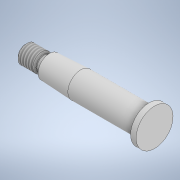
# Autodesk Inventor part: Палец_ребрышко
Saved by Autodesk Inventor 2021 (Build 250183000, 183)
## iProperties
Created: 2023-04-14
Part Number: Палец_ребрышко
Material: Типовые
Document SubType Name: Modeling
Designer: gdevc
Density: 1 g/cm^3
Appearance: По умолчанию
Author: gdevc
Autodesk Inventor part; units mm, degrees
ref_plane "YZ Plane" through (0, 0, 0) normal (1, 0, 0) x (0, 1, 0)
ref_plane "XZ Plane" through (0, 0, 0) normal (0, 1, 0) x (-1, 0, 0)
ref_plane "XY Plane" through (0, 0, 0) normal (0, 0, 1) x (1, 0, 0)
sketch "Эскиз1" plane through (0, 0, 0) normal (0, 0, 1) x (1, 0, 0)
  line L0 (0, 0) -> (0, 5)
  line L1 (0, 5) -> (10, 5)
  line L2 (10, 5) -> (10, 4)
  line L3 (10, 4) -> (13, 4)
  line L4 (13, 4) -> (13, 6.15)
  line L5 (13, 6.15) -> (30, 7)
  line L6 (30, 7) -> (67, 7)
  line L7 (67, 7) -> (67, 10)
  line L8 (67, 10) -> (70, 10)
  line L9 (70, 10) -> (70, 0)
  line L10 (0, 0) -> (70, 0)
  dimension "d0" = 10
  dimension "d1" = 12.3
  dimension "d2" = 14
  dimension "d3" = 10
  dimension "d4" = 3
  dimension "d5" = 20
  dimension "d6" = 8
  dimension "d7" = 60
  dimension "d8" = 3
  dimension "d9" = 20
  constraints: 22 end point, 5 perpendicular, 4 vertical, 1 horizontal
  measures "d0" diameter of L1 L10
  measures "d1" diameter of L4.end L10
  measures "d2" diameter of L5.end L10
  measures "d3" distance of L0.end L1.end
  measures "d4" distance of L2.end L3.end
  measures "d5" distance from line of L5.end L2
  measures "d6" diameter of L3 L10
  measures "d7" distance between parallel lines of L9 L2
  measures "d8" distance between parallel lines of L9 L7
  measures "d9" diameter of L8 L10
revolve "Вращение1" add sketch "Эскиз1" angle 360 about axis through (0, 0, 0) along (1, 0, 0)
thread "Резьба1" size "M10x1.5" class "6g" standard "ISO Metric profile" length 18
chamfer "Фаска1" distance 1 angle 45 2 edges at (0, -5, 0) (10, -5, 0)
fillet "Сопряжение1" radius 0.5 2 edges at (10, -4.0001, 0) (10, -4, 0)
fillet "Сопряжение2" radius 1 1 edges at (13, -4, 0)
